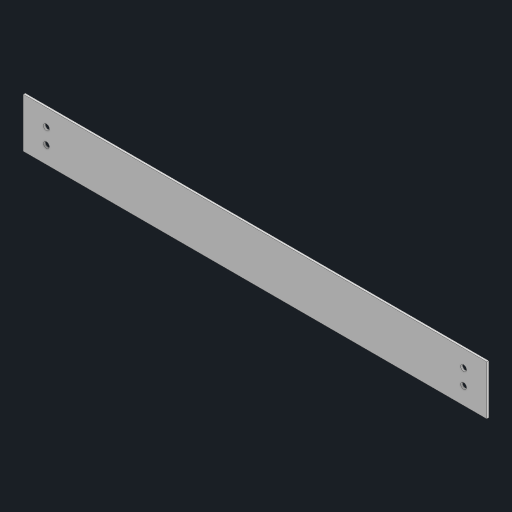
# Autodesk Inventor part: skirtback
Saved by Autodesk Inventor 2023 (Build 270158000, 158)
## iProperties
Created: 2023-04-10
Part Number: skirtback
Material: Generic
Document SubType Name: Modeling
Designer: Windows Macbook
Density: 1 g/cm^3
Appearance: Default
Author: Windows Macbook
Autodesk Inventor part; units mm, degrees
ref_plane "YZ Plane" through (0, 0, 0) normal (1, 0, 0) x (0, 1, 0)
ref_plane "XZ Plane" through (0, 0, 0) normal (0, 1, 0) x (-1, 0, 0)
ref_plane "XY Plane" through (0, 0, 0) normal (0, 0, 1) x (1, 0, 0)
sketch "Sketch1" plane through (0, 0, 0) normal (0, 0, 1) x (1, 0, 0)
  line L0 (0, 0) -> (381, 0)
  line L1 (381, 0) -> (381, 40.64)
  line L2 (381, 40.64) -> (0, 40.64)
  line L3 (0, 40.64) -> (0, 0)
  dimension "d0" = 381
  dimension "d1" = 40.64
  constraints: 8 end point, 2 parallel, 1 horizontal, 1 perpendicular
  measures "d0" distance of L2.end L1.end
  measures "d1" distance of L1.end L0.end
extrude "Extrusion1" add sketch "Sketch1" along normal blind 1.5875
sketch "Sketch2" plane through (0, 0, 1.5875) normal (0, 0, 1) x (1, 0, 0)
  line L0 (0, 40.64) -> (0, 0) projected
  line L1 (0, 0) -> (40.64, 40.64)
  line L2 (381, 40.64) -> (0, 40.64) projected
  line L3 (0, 0) -> (57.4736, 0) construction
  line L4 (40.64, 40.64) -> (0, 40.64)
  line L5 (0, 40.64) -> (20.32, 20.32)
  line L6 (0, 20.32) -> (19.05, 20.32)
  line L7 (19.05, 20.32) -> (19.05, 26.67)
  line L8 (19.05, 26.67) -> (19.05, 13.97)
  line L9 (381, 0) -> (381, 40.64) projected
  line L10 (381, 0) -> (340.36, 40.64)
  line L11 (381, 0) -> (438.4736, 0) construction
  line L12 (340.36, 40.64) -> (381, 40.64)
  line L13 (381, 40.64) -> (360.68, 20.32)
  line L14 (381, 20.32) -> (361.95, 20.32)
  line L15 (361.95, 20.32) -> (361.95, 26.67)
  line L16 (361.95, 26.67) -> (361.95, 13.97)
  dimension "d4" = 45
  dimension "d5" = 45
  dimension "d6" = 19.05
  dimension "d7" = 6.35
  dimension "d8" = 12.7
  dimension "d9" = 135
  dimension "d10" = 19.05
  dimension "d11" = 6.35
  dimension "d12" = 12.7
  dimension "d13" = 0
  constraints: 28 end point, 4 coincident, 4 horizontal, 4 midpoint, 3 collinear, 3 point on line, 2 equal length, 2 perpendicular
  measures "d4" angle of L3 L1
  measures "d5" angle of L5 L4
  measures "d6" distance of L6.start L6.end
  measures "d7" distance of L6.end L7.end
  measures "d8" distance of L7.end L8.end
  measures "d9" angle of L11 L10
  measures "d10" distance of L14.start L14.end
  measures "d11" distance of L14.end L15.end
  measures "d12" distance of L15.end L16.end
  measures "d13" distance between parallel lines of L16 L15
hole "Hole1" at (19.05, 13.97, 1.5875) at (19.05, 26.67, 1.5875) at (361.95, 26.67, 1.5875) at (361.95, 13.97, 1.5875) direction (0, 0, -1) diameter 4.7625 end through all
body "Solid1"
